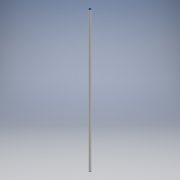
# Autodesk Inventor part: axis_r1
Saved by Autodesk Inventor 2018 (Build 220112000, 112)
## iProperties
Created: 2018-04-20
Part Number: axis_r1
Material: アルミニウム 6061
Document SubType Name: Modeling
Designer: ku_sk
Density: 2.7 g/cm^3
Appearance: アルミニウム - フラット
Mass: 222.576 g
Surface Area: 825.611 cm^2
Volume: 82.4354 cm^3
Author: ku_sk
Autodesk Inventor part; units mm, degrees
ref_plane "YZ Plane" through (0, 0, 0) normal (1, 0, 0) x (0, 1, 0)
ref_plane "XZ Plane" through (0, 0, 0) normal (0, 1, 0) x (-1, 0, 0)
ref_plane "XY Plane" through (0, 0, 0) normal (0, 0, 1) x (1, 0, 0)
sketch "スケッチ1" plane through (0, 0, 0) normal (0, 0, 1) x (1, 0, 0)
  circle A0 centre (0, 0) radius 6
  circle A1 centre (0, 0) radius 4
  dimension "d0" = 2
  dimension "d1" = 12
  constraints: 2 centre point, 2 coincident
  measures "d0" radial gap between concentric circles of A1 A0
  measures "d1" diameter of A0
extrude "押し出し1" add sketch "スケッチ1" along normal mid plane 946
